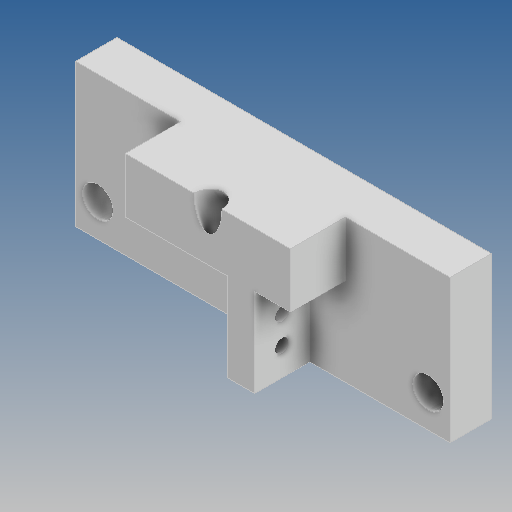
# Autodesk Inventor part: 0008-30-014
Saved by Autodesk Inventor 2020 (Build 240168000, 168)
## iProperties
Created: 2021-06-01
Part Number: 0008-30-014
Material: Generic
Document SubType Name: Modeling
Designer: Iulian Bors
Density: 1 g/cm^3
Appearance: Default
Author: Iulian Bors
Subject: 014
Autodesk Inventor part; units mm, degrees
ref_plane "YZ Plane" through (0, 0, 0) normal (1, 0, 0) x (0, 1, 0)
ref_plane "XZ Plane" through (0, 0, 0) normal (0, 1, 0) x (-1, 0, 0)
sketch "Sketch1" plane through (0, 0, 0) normal (0, 0, 1) x (1, 0, 0)
  line L0 (-68, 26) -> (68, 26)
  line L1 (68, 26) -> (68, -26)
  line L2 (68, -26) -> (-68, -26)
  line L3 (-68, -26) -> (-68, 26)
  point P0 (0, 0)
  point P1 (-68, 0)
  point P2 (0, 26)
  dimension "d0" = 136
  dimension "d1" = 52
  constraints: 8 end point, 2 midpoint, 2 parallel, 1 horizontal, 1 horizontal alignment, 1 perpendicular, 1 vertical alignment
  measures "d0" distance of L0.start L0.end
  measures "d1" distance of L2.end L0.start
extrude "Extrusion1" add sketch "Sketch1" along normal blind 15
sketch "Sketch9" plane through (0, 0, 15) normal (0, 0, 1) x (1, 0, 0)
  circle A0 centre (-60, -14.25) radius 4 projected
  line L0 (188.1551, -73.0673) -> (-511.8449, -73.0673) projected
  circle A1 centre (60, -14.25) radius 4 projected
  point P0 (0, 0)
hole "Hole3" at (-60, -14.25, 15) at (60, -14.25, 15) direction (0, 0, -1) diameter 11 end through all
sketch "Sketch10" plane through (0, 0, 15) normal (0, 0, 1) x (1, 0, 0)
  line L0 (30, 6) -> (-30, 6)
  line L1 (-30, 6) -> (-30, 26)
  line L2 (-30, 26) -> (30, 26)
  line L3 (30, 26) -> (30, 6)
  line L4 (-68, -26) -> (68, -26) projected
  line L5 (68, 26) -> (-68, 26) projected
  point P0 (0, 0)
  point P1 (0, 6)
  dimension "d47" = 60
  dimension "d56" = 20
  constraints: 8 end point, 2 parallel, 1 collinear, 1 horizontal, 1 midpoint, 1 perpendicular, 1 vertical alignment
  measures "d47" distance between parallel lines of L1 L3
  measures "d56" distance of L2.end L0.start
extrude "Extrusion6" add sketch "Sketch10" along normal blind 20
ref_plane "Work Plane1" through (-30, 6, 35) normal (0, -0.8660254, -0.5) x (1, 0, 0)
sketch "Sketch11" plane through (-30, 6, 35) normal (0, -0.8660254, -0.5) x (1, 0, 0)
  circle A0 centre (30, -10) radius 5
  line L0 (0, 0) -> (60, 0) projected
  point P0 (30, -27.3109)
  point P1 (30, 0)
  dimension "d52" = 10
  dimension "d53" = 10
  constraints: 1 centre point, 1 midpoint, 1 vertical alignment
  measures "d52" diameter of A0
  measures "d53" distance from line of A0.centre L0
extrude "Extrusion7" cut sketch "Sketch11" against normal blind 33
sketch "Sketch12" plane through (0, 11, 26.3397) normal (0, 0.8660254, 0.5) x (1, 0, 0)
  circle A0 centre (0, 0) radius 5 projected
  point P0 (0, 17.3109)
extrude "Extrusion8" cut sketch "Sketch12" against normal up to surface surface through (-30, 6, 15) normal (0, -1, 0)
sketch "Sketch13" plane through (0, 0, 15) normal (0, 0, 1) x (1, 0, 0)
  line L0 (17, -26) -> (7, -26)
  line L1 (7, -26) -> (7, 6)
  line L2 (7, 6) -> (17, 6)
  line L3 (17, 6) -> (17, -26)
  line L4 (-30, 6) -> (30, 6) projected
  line L5 (-68, -26) -> (68, -26) projected
  ellipse E0 centre (0, 26) end of major axis (0, 36) minor radius 5 (-5, 26) -> (5, 26) ccw projected
  line L6 (5, 6) -> (-5, 6) projected
  point P0 (0, 0)
  dimension "d59" = 10
  dimension "d62" = 2
  constraints: 8 end point, 2 collinear, 2 parallel, 1 horizontal, 1 perpendicular, 1 other
  measures "d59" distance of L0.start L0.end
  measures "d62" distance from line of L6.start L1
extrude "Extrusion9" add sketch "Sketch13" along normal up to surface (20 mm away)
sketch "Sketch14" plane through (7, -26, 15) normal (-1, 0, 0) x (0, 0, 1)
  line L0 (0, 0) -> (20, 0) projected
  point P0 (-15, 26)
  point P1 (10, 10)
  point P2 (10, 20)
  point P3 (10, 0)
  dimension "d65" = 10
  dimension "d66" = 10
  constraints: 2 vertical alignment, 1 midpoint
  measures "d65" distance from line of point (10, 10) L0
  measures "d66" distance of point (10, 20) point (10, 10)
hole "Hole4" at (7, -16, 25) at (7, -6, 25) direction (1, 0, 0) diameter 5 end through all
body "Solid1"
